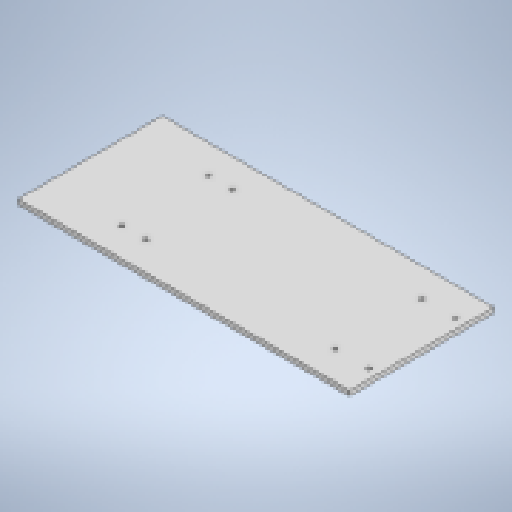
# Autodesk Inventor part: acrylic_side
Saved by Autodesk Inventor 2026.1 (Build 301233000, 233)
## iProperties
Created: 2026-05-13
Part Number: acrylic_side
Material: Generic
Document SubType Name: Modeling
Designer: chris
Density: 1 g/cm^3
Appearance: Default
Author: chris
Autodesk Inventor part; units mm, degrees
ref_plane "YZ Plane" through (0, 0, 0) normal (1, 0, 0) x (0, 1, 0)
ref_plane "XZ Plane" through (0, 0, 0) normal (0, 1, 0) x (-1, 0, 0)
ref_plane "XY Plane" through (0, 0, 0) normal (0, 0, 1) x (1, 0, 0)
sketch "Sketch1" plane through (0, 0, 0) normal (0, 1, 0) x (-1, 0, 0)
  line L0 (172.5, 75) -> (-172.5, 75)
  line L1 (-172.5, 75) -> (-172.5, -75)
  line L2 (-172.5, -75) -> (172.5, -75)
  line L3 (172.5, -75) -> (172.5, 75)
  line L4 (172.5, 75) -> (-172.5, -75) construction
  line L5 (-172.5, 75) -> (172.5, -75) construction
  point P0 (0, 0)
  dimension "d0" = 345
  dimension "d1" = 150
  constraints: 12 end point, 2 midpoint, 2 parallel, 1 horizontal, 1 perpendicular
  measures "d0" distance of L2.end L1.end
  measures "d1" distance of L1.end L0.end
extrude "Extrusion1" add sketch "Sketch1" along normal blind 5
sketch "Sketch2" plane through (0, 0, 0) normal (0, -1, 0) x (1, 0, 0)
  circle A0 centre (162.5, 45) radius 2.05 projected
  circle A1 centre (162.5, -45) radius 2.05 projected
  circle A2 centre (127.5, 45) radius 2.05 projected
  circle A3 centre (127.5, -45) radius 2.05 projected
  line L0 (172.5, -75) -> (47.5, -75) projected
  line L1 (47.5, -75) -> (47.5, -55) projected
  line L2 (117.5, -55) -> (47.5, -55) projected
  line L3 (117.5, -55) -> (117.5, 75) projected
  line L4 (117.5, 75) -> (172.5, 75) projected
  line L5 (172.5, -75) -> (172.5, 75) projected
  line L6 (-104.55, -45) -> (-104.55, 60) projected
  line L7 (-104.55, 60) -> (-132, 60) projected
  line L8 (-132, 75) -> (-132, 60) projected
  line L9 (-132, 75) -> (-32, 75) projected
  line L10 (-32, 60) -> (-32, 75) projected
  line L11 (-32, 60) -> (-59.45, 60) projected
  line L12 (-59.45, 60) -> (-59.45, -45) projected
  arc A4 (-59.45, -45) -> (-54.45, -50) centre (-54.45, -45) ccw projected
  line L13 (-32, -50) -> (-54.45, -50) projected
  line L14 (-32, -75) -> (-32, -50) projected
  line L15 (-59.45, -75) -> (-32, -75) projected
  line L16 (-59.45, -75) -> (-59.45, -65) projected
  line L17 (-59.45, -65) -> (-104.55, -65) projected
  line L18 (-104.55, -65) -> (-104.55, -75) projected
  line L19 (-132, -75) -> (-104.55, -75) projected
  line L20 (-132, -50) -> (-132, -75) projected
  line L21 (-109.55, -50) -> (-132, -50) projected
  arc A5 (-109.55, -50) -> (-104.55, -45) centre (-109.55, -45) ccw projected
  circle A6 centre (-94.5, 45) radius 2.05 projected
  circle A7 centre (-69.5, -45) radius 2.05 projected
  circle A8 centre (-69.5, 45) radius 2.05 projected
  circle A9 centre (-94.5, -45) radius 2.05 projected
  circle A10 centre (162.5, 45) radius 2
  circle A11 centre (162.5, -45) radius 2
  circle A12 centre (127.5, 45) radius 2
  circle A13 centre (127.5, -45) radius 2
  circle A14 centre (-69.5, 45) radius 2
  circle A15 centre (-69.5, -45) radius 2
  circle A16 centre (-94.5, 45) radius 2
  circle A17 centre (-94.5, -45) radius 2
  point P0 (0, 0)
  dimension "d4" = 4
  dimension "d5" = 4
  dimension "d6" = 4
  dimension "d7" = 4
  dimension "d8" = 4
  dimension "d9" = 4
  dimension "d10" = 4
  dimension "d11" = 4
  constraints: 8 centre point, 8 coincident
  measures "d4" diameter of A10
  measures "d5" diameter of A11
  measures "d6" diameter of A12
  measures "d7" diameter of A13
  measures "d8" diameter of A14
  measures "d9" diameter of A15
  measures "d10" diameter of A16
  measures "d11" diameter of A17
extrude "Extrusion2" cut sketch "Sketch2" against normal blind 5 contours A10 | A11 | A12 | A13 | A14 | A15 | A16 | A17
body "Solid1"
